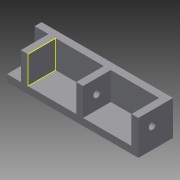
# Autodesk Inventor part: corner
Saved by Autodesk Inventor 2013 (Build 170138000, 138)
## iProperties
Created: 2013-02-01
Part Number: corner
Material: Generic
Document SubType Name: Modeling
Designer: Brad
Density: 1 g/cm^3
Author: Brad
Autodesk Inventor part; units mm, degrees
ref_plane "YZ Plane" through (0, 0, 0) normal (1, 0, 0) x (0, 1, 0)
ref_plane "XZ Plane" through (0, 0, 0) normal (0, 1, 0) x (-1, 0, 0)
ref_plane "XY Plane" through (0, 0, 0) normal (0, 0, 1) x (1, 0, 0)
sketch "Sketch1" plane through (0, 0, 0) normal (0, 0, 1) x (1, 0, 0)
  line L0 (-11.658, 3.4387) -> (-11.658, -28.3113)
  line L1 (-11.658, 3.4387) -> (108.992, 3.4387)
  line L2 (108.992, 3.4387) -> (108.992, -28.3113)
  line L3 (108.992, -28.3113) -> (-11.658, -28.3113)
  point P0 (0, 0)
  dimension "d0" = 31.75
  dimension "d1" = 120.65
  dimension "d2" = 31.75
  constraints: 8 end point, 2 perpendicular, 1 vertical
  measures "d0" distance of L0.start L0.end
  measures "d1" distance of L0.start L1.end
  measures "d2" distance of L1.end L2.end
extrude "Extrusion1" add sketch "Sketch1" along normal blind 6.35
sketch "Sketch2" plane through (0, 0, 6.35) normal (0, 0, 1) x (1, 0, 0)
  line L0 (-11.658, 3.4387) -> (-11.658, -28.3113) projected
  line L1 (-11.658, -28.3113) -> (108.992, -28.3113) projected
  line L2 (108.992, -28.3113) -> (108.992, 3.4387) projected
  line L3 (-11.658, -28.3113) -> (-11.658, -21.9613)
  line L4 (-11.658, -21.9613) -> (108.992, -21.9613)
  line L5 (108.992, -28.3113) -> (-11.658, -28.3113)
  point P0 (0, 0)
  dimension "d5" = 6.35
  constraints: 6 end point, 2 point on line, 1 collinear, 1 perpendicular
  measures "d5" distance of L0.end L3.end
extrude "Extrusion2" add sketch "Sketch2" along normal blind 25.4
sketch "Sketch3" plane through (-11.658, -21.9613, 6.35) normal (0, 1, 0) x (1, 0, 0)
  line L0 (0, 0) -> (120.65, 0) projected
  line L1 (120.65, -25.4) -> (0, -25.4) projected
  line L2 (120.65, 0) -> (120.65, -25.4) projected
  line L3 (0, -25.4) -> (12.7, -25.4)
  line L4 (12.7, -25.4) -> (12.7, 0)
  line L5 (12.7, 0) -> (19.05, 0)
  line L6 (19.05, 0) -> (19.05, -25.4)
  line L7 (19.05, -25.4) -> (12.7, -25.4)
  line L8 (19.05, -25.4) -> (63.5, -25.4)
  line L9 (63.5, -25.4) -> (63.5, 0)
  line L10 (63.5, 0) -> (69.85, 0)
  line L11 (69.85, 0) -> (69.85, -25.4)
  line L12 (69.85, -25.4) -> (63.5, -25.4)
  line L13 (69.85, -25.4) -> (114.3, -25.4)
  line L14 (114.3, -25.4) -> (114.3, 0)
  line L15 (120.65, 0) -> (114.3, 0)
  line L16 (120.65, 0) -> (120.65, -25.4)
  line L17 (114.3, -25.4) -> (120.65, -25.4)
  point P0 (11.658, 6.35)
  dimension "d8" = 12.7
  dimension "d9" = 6.35
  dimension "d10" = 25.4
  dimension "d11" = 44.45
  dimension "d12" = 6.35
  dimension "d13" = 25.4
  dimension "d14" = 44.45
  constraints: 30 end point, 10 point on line, 5 perpendicular, 3 collinear
  measures "d8" distance of L1.end L3.end
  measures "d9" distance of L4.end L5.end
  measures "d10" distance of L5.end L6.end
  measures "d11" distance of L6.end L8.end
  measures "d12" distance of L9.end L10.end
  measures "d13" distance of L10.end L11.end
  measures "d14" distance of L11.end L13.end
extrude "Extrusion3" add sketch "Sketch3" along normal blind 25.4 contours L0 L6 L1 L4 | L0 L11 L1 L9 | L0 L2 L1 L14
sketch "Sketch4" plane through (7.392, -21.9613, 31.75) normal (1, 0, 0) x (0, 0, -1)
  line L0 (25.4, 0) -> (0, 0) projected
  line L1 (25.4, 25.4) -> (25.4, 0) projected
  line L2 (0, 25.4) -> (25.4, 25.4) projected
  line L3 (0, 0) -> (0, 25.4) projected
  point P0 (31.75, 21.9613)
sketch "Sketch5" plane through (108.992, -28.3113, 0) normal (1, 0, 0) x (0, 0, -1)
  line L0 (-31.75, 0) -> (-31.75, 31.75) projected
  line L1 (-31.75, 31.75) -> (-31.75, 19.05)
  line L2 (-31.75, 19.05) -> (-19.05, 19.05)
  circle A0 centre (-19.05, 19.05) radius 3.175
  point P0 (0, 28.3113)
  dimension "d17" = 12.7
  dimension "d18" = 12.7
  dimension "d19" = 6.35
  constraints: 4 end point, 1 centre point, 1 coincident, 1 perpendicular, 1 point on line
  measures "d17" distance of L0.end L1.end
  measures "d18" distance of L1.end L2.end
  measures "d19" diameter of A0
extrude "Extrusion4" cut sketch "Sketch5" against normal blind 76.2
body "Solid1"
